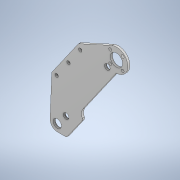
# Autodesk Inventor part: FrontLink_frame
Saved by Autodesk Inventor 2020 (Build 240168000, 168)
## iProperties
Created: 2021-10-03
Part Number: FrontLink_frame
Material: GFRP
Document SubType Name: Modeling
Designer: Masato Kubotera
Density: 1.75 g/cm^3
Appearance: 滑らか - 淡い灰色
Description: GFRP T2
Mass: 10.1997 g
Surface Area: 66.8834 cm^2
Volume: 5.82838 cm^3
Author: Masato Kubotera
Autodesk Inventor part; units mm, degrees
ref_plane "YZ Plane" through (0, 0, 0) normal (1, 0, 0) x (0, 1, 0)
ref_plane "XZ Plane" through (0, 0, 0) normal (0, 1, 0) x (-1, 0, 0)
ref_plane "XY Plane" through (0, 0, 0) normal (0, 0, 1) x (1, 0, 0)
derived "Link_basis.ipt"
sketch "スケッチ1" plane through (0, 0, 0) normal (0, 0, 1) x (1, 0, 0)
  circle A0 centre (0, 0) radius 6
  circle A1 centre (-57.3576, -81.9152) radius 4
  arc A2 (-64.3515, -81.6228) -> (-57.3576, -88.9152) centre (-57.3576, -81.9152) ccw
  arc A3 (-0.1434, -10.9991) -> (-4.5598, 10.0104) centre (0, 0) ccw
  line L0 (-61.4483, -42.4277) -> (-35.6374, -5.5658) construction
  line L1 (-35.6374, -5.5658) -> (-31.5416, -8.4337) construction
  line L2 (-31.5416, -8.4337) -> (-57.3525, -45.2955) construction
  line L3 (-57.3525, -45.2955) -> (-61.4483, -42.4277) construction
  line L4 (-61.4483, -42.4277) -> (-31.5416, -8.4337) construction
  line L5 (-35.6374, -5.5658) -> (-57.3525, -45.2955) construction
  line L6 (-59.4004, -43.8616) -> (-33.5895, -6.9998) construction
  circle A4 centre (-57.9665, -41.8137) radius 1.6
  circle A5 centre (-46.495, -25.4307) radius 1.6
  line L7 (-48.5428, -23.9967) -> (-44.4471, -26.8646) construction
  circle A6 centre (-35.0234, -9.0476) radius 1.6
  line L8 (-62.677, -41.5673) -> (-36.8661, -4.7054)
  line L9 (-36.8661, -4.7054) -> (-4.5598, 10.0104)
  line L10 (-62.677, -41.5673) -> (-64.3515, -81.6228)
  line L11 (-32.3614, -57.0111) -> (-0.1434, -10.9991)
  line L12 (0, 0) -> (32, 0) construction
  line L13 (32, 0) -> (32, 20) construction
  circle A7 centre (32, 20) radius 4
  arc A8 (38.9218, 15.1533) -> (32, 28.45) centre (32, 20) ccw
  line L14 (32, 20) -> (32, 37) construction
  circle A9 centre (32, 37) radius 4 construction
  circle A10 centre (32, 37) radius 8.45 construction
  line L15 (-57.3576, -81.9152) -> (0, 0) construction
  circle A11 centre (0, 0) radius 8.5 construction
  circle A12 centre (6.0104, 6.0104) radius 1.4
  circle A13 centre (32, 20) radius 7 construction
  arc A14 (-64.3515, -81.6228) -> (-53.3426, -76.1811) centre (-57.3576, -81.9152) ccw construction
  line L16 (-51.6236, -85.9302) -> (-33.7808, -60.4482)
  line L17 (38.9218, 15.1533) -> (-18.4358, -66.7619)
  line L18 (32, 20) -> (-25.3576, -61.9152) construction
  circle A15 centre (-25.3576, -61.9152) radius 4
  circle A16 centre (-25.3576, -61.9152) radius 8 construction
  arc A17 (-0.0917, -11.0996) -> (11.1, 0) centre (0, 0) ccw
  line L19 (25.0782, 24.8467) -> (10.3989, 3.8825)
  line L20 (-0.0917, -11.0996) -> (-32.2795, -57.0685)
  arc A18 (-32.2795, -57.0685) -> (-18.4358, -66.7619) centre (-25.3576, -61.9152) ccw
  arc A19 (-32.3614, -57.0111) -> (-32.5799, -66.4914) centre (-25.3576, -61.9152) ccw
  line L21 (-6.0104, 6.0104) -> (0, 0) construction
  circle A20 centre (-6.0104, 6.0104) radius 1.4
  circle A21 centre (-6.0104, -6.0104) radius 1.4
  circle A22 centre (6.0104, -6.0104) radius 1.4
  line L22 (-12.2888, -46.6506) -> (2.0506, -26.1718) construction
  line L23 (2.0506, -26.1718) -> (6.1464, -29.0397) construction
  line L24 (6.1464, -29.0397) -> (-8.193, -49.5185) construction
  line L25 (-8.193, -49.5185) -> (-12.2888, -46.6506) construction
  line L26 (-12.2888, -46.6506) -> (6.1464, -29.0397) construction
  line L27 (2.0506, -26.1718) -> (-8.193, -49.5185) construction
  line L28 (4.0985, -27.6058) -> (-10.2409, -48.0846) construction
  line L29 (-5.1191, -36.4112) -> (-1.0233, -39.2791) construction
  circle A23 centre (2.6646, -29.6537) radius 1.6
  circle A24 centre (-8.8069, -46.0367) radius 1.6
  line L30 (7.185, 8.4608) -> (11.1, 14.052)
  line L31 (32, 28.45) -> (21.1816, 28.45)
  arc A25 (32, 28.45) -> (25.0782, 24.8467) centre (32, 20) ccw construction
  line L32 (-32.5799, -66.4914) -> (-48.2812, -88.9152)
  line L33 (-57.3576, -88.9152) -> (-48.2812, -88.9152)
  arc A26 (-57.3576, -88.9152) -> (-51.6236, -85.9302) centre (-57.3576, -81.9152) ccw construction
  line L34 (10.253, -29.3449) -> (-8.8388, -10.253) construction
  line L35 (-8.8388, -10.253) -> (10.253, 8.8388) construction
  line L36 (10.253, 8.8388) -> (29.3449, -10.253) construction
  line L37 (29.3449, -10.253) -> (10.253, -29.3449) construction
  line L38 (10.253, -29.3449) -> (10.253, 8.8388) construction
  line L39 (-8.8388, -10.253) -> (29.3449, -10.253) construction
  line L40 (0.7071, -0.7071) -> (19.799, -19.799) construction
  circle A27 centre (-8.8388, -10.253) radius 2.699
  circle A28 centre (-6.0104, -6.0104) radius 2.4 construction
  line L41 (-42.1647, -109.0339) -> (-64.2818, -93.5473) construction
  line L42 (-64.2818, -93.5473) -> (-48.7952, -71.4302) construction
  line L43 (-48.7952, -71.4302) -> (-26.6781, -86.9168) construction
  line L44 (-26.6781, -86.9168) -> (-42.1647, -109.0339) construction
  line L45 (-42.1647, -109.0339) -> (-48.7952, -71.4302) construction
  line L46 (-64.2818, -93.5473) -> (-26.6781, -86.9168) construction
  line L47 (-56.5385, -82.4888) -> (-34.4214, -97.9753) construction
  circle A29 centre (-48.7952, -71.4302) radius 2.699
  line L48 (11.1, 0) -> (11.1, 14.052)
  line L49 (11.1, 14.052) -> (21.1816, 28.45)
  arc A30 (11.1, 0) -> (7.185, 8.4608) centre (0, 0) ccw construction
  line L50 (0, 0) -> (6.0104, 6.0104)
  line L51 (0.6167, -28.2197) -> (4.7125, -31.0876) construction
  line L52 (13.5222, -9.7888) -> (-0.8172, -30.2676) construction
  line L53 (3.2785, -33.1355) -> (17.6179, -12.6567) construction
  line L54 (6.3525, -20.0282) -> (10.4482, -22.8961) construction
  line L55 (17.6179, -12.6567) -> (13.5222, -9.7888) construction
  circle A31 centre (14.1361, -13.2706) radius 1.6
  line L56 (-0.8172, -30.2676) -> (3.2785, -33.1355) construction
  point P0 (-3.0712, -37.8452)
  point P1 (-64.3015, -81.0305)
  point P2 (10.253, -10.253)
  point P3 (-45.4799, -90.2321)
  dimension "d5" = 27
  dimension "d6" = 27
  dimension "d9" = 10
  dimension "d12" = 4.8
  dimension "d13" = 27
  dimension "d14" = 27
  dimension "d17" = 0
  dimension "d18" = 1
  dimension "d19" = 1
  dimension "d20" = 5.398
  dimension "d21" = 5.398
  measures "d5" distance of L35.end L36.end
  measures "d6" distance of L34.end L35.end
  measures "d9" angle of L35 L15
  measures "d12" diameter of A28
  measures "d13" distance of L42.end L43.end
  measures "d14" distance of L41.end L42.end
  measures "d17" angle of L15 L42
  measures "d18" distance from line of point (0, 0) L35
  measures "d19" distance from line of A1.centre L42
  measures "d20" diameter of A27
  measures "d21" diameter of A29
extrude "押し出し1" add sketch "スケッチ1" along normal blind 2 contours L10 L8 L9 A3 L11 A19 L32 L33 A2
fillet "フィレット1" radius 2 3 edges at (-36.8661, -4.7054, 1) (-62.677, -41.5673, 1) (-0.1434, -10.9991, 1)
fillet "フィレット2" radius 2 2 edges at (-32.5799, -66.4914, 1) (-48.2812, -88.9152, 1)
equation "\"d21\" = d20"
